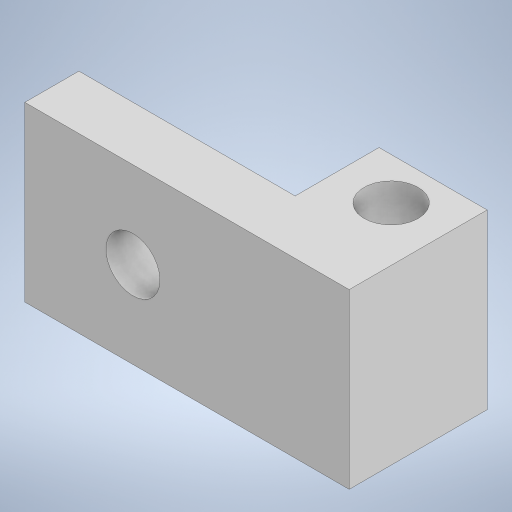
# Autodesk Inventor part: cover mount LR v02
Saved by Autodesk Inventor 2023 (Build 270158000, 158)
## iProperties
Created: 2024-06-30
Part Number: cover mount LR v02
Material: Generic
Document SubType Name: Modeling
Designer: Akramilab
Density: 1 g/cm^3
Appearance: Default
Author: Akramilab
Autodesk Inventor part; units mm, degrees
ref_plane "YZ Plane" through (0, 0, 0) normal (1, 0, 0) x (0, 1, 0)
ref_plane "XZ Plane" through (0, 0, 0) normal (0, 1, 0) x (-1, 0, 0)
ref_plane "XY Plane" through (0, 0, 0) normal (0, 0, 1) x (1, 0, 0)
sketch "Sketch1" plane through (0, 0, 0) normal (0, 0, 1) x (1, 0, 0)
  line L0 (0, 0) -> (20, 0)
  line L1 (20, 0) -> (20, -16)
  line L2 (20, -16) -> (0, -16)
  line L3 (0, -16) -> (0, 0)
  circle A0 centre (10, -8) radius 2.5
  dimension "d0" = 20
  dimension "d1" = 16
  dimension "d2" = 8
  dimension "d3" = 10
  dimension "d4" = 5
  constraints: 8 end point, 2 parallel, 1 centre point, 1 coincident, 1 horizontal, 1 perpendicular
  measures "d0" distance of L1.end L2.end
  measures "d1" distance of L0.end L1.end
  measures "d2" distance from line of point (10, -8) L2
  measures "d3" distance from line of L1 point (10, -8)
  measures "d4" diameter of A0
extrude "Extrusion1" add sketch "Sketch1" along normal blind 5
sketch "Sketch2" plane through (0, 0, 0) normal (0, 1, 0) x (1, 0, 0)
  line L0 (20, 0) -> (20, -5) projected
  line L1 (20, 0) -> (30, 0)
  line L2 (30, 0) -> (30, 7.76)
  line L3 (30, 7.76) -> (20, 7.76)
  line L4 (20, 7.76) -> (20, 0)
  line L5 (20, -5) -> (30, -5)
  line L6 (30, -5) -> (30, 0)
  line L7 (30, 0) -> (20, 0)
  line L8 (20, 0) -> (20, -5)
  circle A0 centre (25, 3.88) radius 2.5
  point P0 (0, 0)
  dimension "d7" = 10
  dimension "d8" = 7.76
  dimension "d9" = 5
  constraints: 16 end point, 4 parallel, 2 horizontal, 2 perpendicular, 1 centre point
  measures "d7" distance of L3.end L2.end
  measures "d8" distance of L2.end L1.end
  measures "d9" diameter of A0
extrude "Extrusion2" add sketch "Sketch2" against normal blind 16
sketch "Sketch3" plane through (0, -16, 0) normal (0, -1, 0) x (1, 0, 0)
  line L0 (30, -7.76) -> (30, 5) projected
  line L1 (0, 0) -> (20, 0) projected
  line L2 (30, -7.76) -> (20, -7.76)
  line L3 (20, -7.76) -> (20, 0)
  line L4 (20, 0) -> (30, 0)
  line L5 (30, 0) -> (30, -7.76)
  constraints: 8 end point, 2 parallel, 1 horizontal, 1 perpendicular
extrude "Extrusion3" add sketch "Sketch3" against normal blind 9
equation "\"d2\" = 0.5 * d1"
equation "\"d3\" = 0.5 * d0"
body "Solid1"
